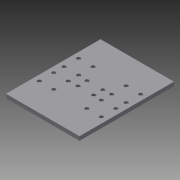
# Autodesk Inventor part: mic6_plate
Saved by Autodesk Inventor 2014 (Build 180170000, 170)
## iProperties
Created: 2014-08-09
Part Number: mic6_plate
Material: Generic
Document SubType Name: Modeling
Designer: Matthew
Density: 1 g/cm^3
Appearance: Default
Author: Matthew
Autodesk Inventor part; units mm, degrees
ref_plane "YZ Plane" through (0, 0, 0) normal (1, 0, 0) x (0, 1, 0)
ref_plane "XZ Plane" through (0, 0, 0) normal (0, 1, 0) x (-1, 0, 0)
ref_plane "XY Plane" through (0, 0, 0) normal (0, 0, 1) x (1, 0, 0)
sketch "Sketch1" plane through (0, 0, 0) normal (0, 1, 0) x (-1, 0, 0)
  line L0 (88.9, 114.3) -> (-88.9, 114.3)
  line L1 (-88.9, 114.3) -> (-88.9, -114.3)
  line L2 (-88.9, -114.3) -> (88.9, -114.3)
  line L3 (88.9, -114.3) -> (88.9, 114.3)
  line L4 (88.9, 114.3) -> (-88.9, -114.3) construction
  line L5 (-88.9, 114.3) -> (88.9, -114.3) construction
  point P0 (0, 0)
  dimension "d0" = 177.8
  dimension "d1" = 228.6
  constraints: 12 end point, 2 midpoint, 2 parallel, 1 horizontal, 1 perpendicular
  measures "d0" distance of L2.end L1.end
  measures "d1" distance of L0.end L1.end
extrude "Extrusion1" add sketch "Sketch1" along normal blind 9.525
sketch "Sketch2" plane through (0, 9.525, 0) normal (0, 1, 0) x (1, 0, 0)
  line L0 (-88.9, 114.3) -> (-88.9, -114.3) projected
  line L1 (-88.9, -114.3) -> (88.9, -114.3) projected
  point P0 (-152.4, 133.35)
  point P1 (-152.4, -133.35)
  point P2 (-133.35, -152.4)
  point P3 (133.35, -152.4)
  point P4 (0, 0)
  point P5 (-63.5, -88.9)
  point P6 (-63.5, -38.1)
  point P7 (-63.5, 12.7)
  point P8 (-63.5, 63.5)
  point P9 (-63.5, 114.3)
  point P10 (-63.5, 165.1)
  point P11 (-38.1, -88.9)
  point P12 (-38.1, -38.1)
  point P13 (-38.1, 12.7)
  point P14 (-38.1, 63.5)
  point P15 (-38.1, 114.3)
  point P16 (-38.1, 165.1)
  point P17 (-12.7, -88.9)
  point P18 (-12.7, -38.1)
  point P19 (-12.7, 12.7)
  point P20 (-12.7, 63.5)
  point P21 (-12.7, 114.3)
  point P22 (-12.7, 165.1)
  point P23 (12.7, -88.9)
  point P24 (12.7, -38.1)
  point P25 (12.7, 12.7)
  point P26 (12.7, 63.5)
  point P27 (12.7, 114.3)
  point P28 (12.7, 165.1)
  point P29 (38.1, -88.9)
  point P30 (38.1, -38.1)
  point P31 (38.1, 12.7)
  point P32 (38.1, 63.5)
  point P33 (38.1, 114.3)
  point P34 (38.1, 165.1)
  point P35 (63.5, -88.9)
  point P36 (63.5, -38.1)
  point P37 (63.5, 12.7)
  point P38 (63.5, 63.5)
  point P39 (63.5, 114.3)
  point P40 (63.5, 165.1)
  point P41 (88.9, -88.9)
  point P42 (88.9, -38.1)
  point P43 (88.9, 12.7)
  point P44 (88.9, 63.5)
  point P45 (88.9, 114.3)
  point P46 (88.9, 165.1)
  point P47 (114.3, -88.9)
  point P48 (114.3, -38.1)
  point P49 (114.3, 12.7)
  point P50 (114.3, 63.5)
  point P51 (114.3, 114.3)
  point P52 (114.3, 165.1)
  point P53 (139.7, -88.9)
  point P54 (139.7, -38.1)
  point P55 (139.7, 12.7)
  point P56 (139.7, 63.5)
  point P57 (139.7, 114.3)
  point P58 (139.7, 165.1)
  point P59 (165.1, -88.9)
  point P60 (165.1, -38.1)
  point P61 (165.1, 12.7)
  point P62 (165.1, 63.5)
  point P63 (165.1, 114.3)
  point P64 (165.1, 165.1)
  point P65 (190.5, -88.9)
  point P66 (190.5, -38.1)
  point P67 (190.5, 12.7)
  point P68 (190.5, 63.5)
  point P69 (190.5, 114.3)
  point P70 (190.5, 165.1)
  point P71 (88.9, -114.3)
  dimension "d8" = 25.4
  dimension "d9" = 25.4
  dimension "d12" = 50.8
  dimension "d15" = 25.4
  constraints: 60 horizontal alignment, 5 vertical alignment, 2 other
  measures "d12" distance of point (-63.5, -88.9) point (-63.5, -38.1)
  measures "d15" distance of point (-63.5, -88.9) point (-38.1, -88.9)
hole "Hole1" [suppressed]
sketch "Sketch3" plane through (0, 9.525, 0) normal (0, 1, 0) x (1, 0, 0)
  line L0 (-88.9, 114.3) -> (-88.9, -114.3) projected
  line L1 (88.9, 114.3) -> (-88.9, 114.3) projected
  line L2 (-81.4996, 55) -> (-81.4996, 5) construction
  line L3 (-81.4996, 5) -> (-33.4996, 5) construction
  line L4 (-33.4996, 5) -> (-33.4996, 55) construction
  line L5 (-33.4996, 55) -> (-81.4996, 55) construction
  line L6 (33.4996, 55) -> (33.4996, 5) construction
  line L7 (33.4996, 5) -> (81.4996, 5) construction
  line L8 (81.4996, 5) -> (81.4996, 55) construction
  line L9 (81.4996, 55) -> (33.4996, 55) construction
  line L10 (-81.4996, -5) -> (-81.4996, -55) construction
  line L11 (-81.4996, -55) -> (-33.4996, -55) construction
  line L12 (-33.4996, -55) -> (-33.4996, -5) construction
  line L13 (-33.4996, -5) -> (-81.4996, -5) construction
  line L14 (33.4996, -5) -> (33.4996, -55) construction
  line L15 (33.4996, -55) -> (81.4996, -55) construction
  line L16 (81.4996, -55) -> (81.4996, -5) construction
  line L17 (81.4996, -5) -> (33.4996, -5) construction
  line L18 (-24, 17.5) -> (24, 17.5) construction
  line L19 (24, 17.5) -> (24, -17.5) construction
  line L20 (24, -17.5) -> (-24, -17.5) construction
  line L21 (-24, -17.5) -> (-24, 17.5) construction
  point P0 (-133.35, 152.4)
  point P1 (-152.4, 133.35)
  point P2 (-152.4, -133.35)
  point P3 (133.35, 152.4)
  point P4 (0, 0)
  point P5 (-74.9996, 47.5)
  point P6 (-39.9996, 47.5)
  point P7 (-74.9996, 12.5)
  point P8 (-39.9996, 12.5)
  point P9 (39.9996, 47.5)
  point P10 (74.9996, 47.5)
  point P11 (39.9996, 12.5)
  point P12 (74.9996, 12.5)
  point P13 (-74.9996, -12.5)
  point P14 (-39.9996, -12.5)
  point P15 (-74.9996, -47.5)
  point P16 (-39.9996, -47.5)
  point P17 (39.9996, -12.5)
  point P18 (74.9996, -12.5)
  point P19 (39.9996, -47.5)
  point P20 (74.9996, -47.5)
  point P21 (0, 17.5)
  point P22 (57.4996, 0)
  point P23 (24, 0)
  point P24 (57.4996, 55)
  point P25 (-18, 11)
  point P26 (20, 11)
  point P27 (-18, -11)
  point P28 (20, -11)
  point P29 (-88.9, -114.3)
  dimension "d27" = 35
  dimension "d30" = 35
  dimension "d33" = 48
  dimension "d34" = 50
  dimension "d35" = 6.5
  dimension "d36" = 6.5
  dimension "d37" = 7.5
  dimension "d38" = 7.5
  dimension "d42" = 114.9992
  dimension "d45" = 60
  dimension "d50" = 48
  dimension "d51" = 35
  dimension "d52" = 6
  dimension "d53" = 6.5
  dimension "d56" = 38
  dimension "d59" = 22
  dimension "d78" = 9.4996
  dimension "d79" = 9.4996
  dimension "d80" = 10
  dimension "d81" = 5
  dimension "d82" = 162.9992
  dimension "d83" = 110
  constraints: 40 end point, 20 vertical alignment, 11 horizontal alignment, 10 parallel, 6 collinear, 3 midpoint, 2 horizontal, 2 perpendicular, 2 vertical, 5 other
  measures "d27" distance of point (-75, 47.5) point (-40, 47.5)
  measures "d30" distance of point (-75, 47.5) point (-75, 12.5)
  measures "d33" distance of L2.end L3.end
  measures "d34" distance of L3.end L4.end
  measures "d35" distance from line of L4 point (-40, 47.5)
  measures "d36" distance from line of L2 point (-75, 47.5)
  measures "d37" distance from line of L5 point (-40, 47.5)
  measures "d38" distance from line of L3 point (-40, 12.5)
  measures "d42" distance of L2.start L6.start
  measures "d45" distance of L2.start L10.start
  measures "d50" distance of L19.end L20.end
  measures "d51" distance of L18.end L19.end
  measures "d52" distance from line of L21 point (-18, 11)
  measures "d53" distance from line of L18 point (-18, 11)
  measures "d56" distance of point (-18, 11) point (20, 11)
  measures "d59" distance of point (-18, 11) point (-18, -11)
  measures "d78" distance between parallel lines of L21 L12
  measures "d79" distance between parallel lines of L14 L19
  measures "d80" distance between parallel lines of L7 L17
  measures "d81" distance from line of point (57.5, 0) L17
  measures "d82" distance between parallel lines of L16 L10
  measures "d83" distance between parallel lines of L15 L9
hole "Hole2" at (-74.9996, 9.525, -47.5) at (-39.9996, 9.525, -47.5) at (-74.9996, 9.525, -12.5) at (-39.9996, 9.525, -12.5) at (74.9996, 9.525, -12.5) at (39.9996, 9.525, -12.5) at (74.9996, 9.525, -47.5) at (39.9996, 9.525, -47.5) at (-39.9996, 9.525, 47.5) at (-74.9996, 9.525, 47.5) at (-39.9996, 9.525, 12.5) at (-74.9996, 9.525, 12.5) at (74.9996, 9.525, 47.5) at (39.9996, 9.525, 47.5) at (74.9996, 9.525, 12.5) at (39.9996, 9.525, 12.5) at (-18, 9.525, -11) at (20, 9.525, -11) at (-18, 9.525, 11) at (20, 9.525, 11) direction (0, -1, 0) diameter 5.5 depth 25.4 tip angle 118
sketch "Sketch4" plane through (0, 9.525, 0) normal (0, 1, 0) x (1, 0, 0)
  circle A0 centre (-18, -11) radius 2.75 projected
  circle A1 centre (-18, 11) radius 2.75 projected
  circle A2 centre (74.9996, -12.5) radius 2.75 projected
  circle A3 centre (74.9996, -47.5) radius 2.75 projected
  circle A4 centre (-39.9996, -12.5) radius 2.75 projected
  circle A5 centre (-39.9996, -47.5) radius 2.75 projected
  circle A6 centre (74.9996, 47.5) radius 2.75 projected
  circle A7 centre (74.9996, 12.5) radius 2.75 projected
  circle A8 centre (-74.9996, 12.5) radius 2.75 projected
  circle A9 centre (-74.9996, 47.5) radius 2.75 projected
  circle A10 centre (-39.9996, 47.5) radius 2.75 projected
  circle A11 centre (-39.9996, 12.5) radius 2.75 projected
  circle A12 centre (39.9996, 12.5) radius 2.75 projected
  circle A13 centre (39.9996, 47.5) radius 2.75 projected
  circle A14 centre (-74.9996, -47.5) radius 2.75 projected
  circle A15 centre (-74.9996, -12.5) radius 2.75 projected
  circle A16 centre (39.9996, -47.5) radius 2.75 projected
  circle A17 centre (39.9996, -12.5) radius 2.75 projected
  circle A18 centre (20, 11) radius 2.75 projected
  circle A19 centre (20, -11) radius 2.75 projected
  point P0 (0, 0)
  constraints: 20 coincident
hole "Hole3" at (-74.9996, 9.525, -47.5) at (-39.9996, 9.525, -47.5) at (-39.9996, 9.525, -12.5) at (-74.9996, 9.525, -12.5) at (-74.9996, 9.525, 12.5) at (-39.9996, 9.525, 12.5) at (-18, 9.525, 11) at (-18, 9.525, -11) at (20, 9.525, -11) at (20, 9.525, 11) at (-74.9996, 9.525, 47.5) at (-39.9996, 9.525, 47.5) at (39.9996, 9.525, -47.5) at (74.9996, 9.525, -47.5) at (74.9996, 9.525, -12.5) at (39.9996, 9.525, -12.5) at (39.9996, 9.525, 12.5) at (74.9996, 9.525, 12.5) at (74.9996, 9.525, 47.5) at (39.9996, 9.525, 47.5) direction (0, -1, 0) diameter 9 depth 5 tip angle 118
equation "\"d30\" = d27"
equation "\"d78\" = d79"
equation "\"d81\" = 0.5 * d80"
body "Solid1"
